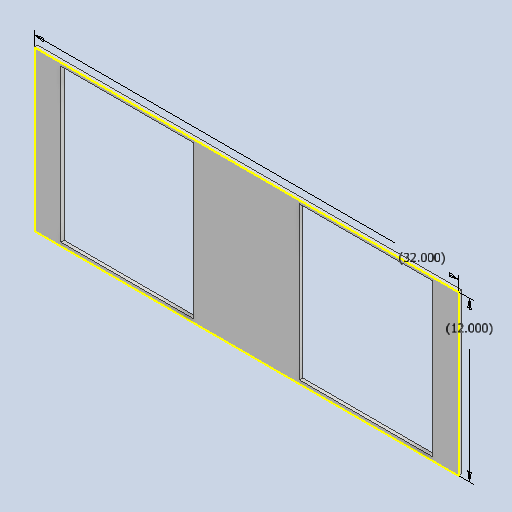
# Autodesk Inventor part: bottom_plywood_Ocampo
Saved by Autodesk Inventor 2023 (Build 270158000, 158)
## iProperties
Created: 2025-02-18
Part Number: bottom_plywood_Ocampo
Material: Generic
Document SubType Name: Modeling
Designer: 1244275
Density: 1 g/cm^3
Appearance: Default
Author: 1244275
Autodesk Inventor part; units mm, degrees
ref_plane "YZ Plane" through (0, 0, 0) normal (1, 0, 0) x (0, 1, 0)
ref_plane "XZ Plane" through (0, 0, 0) normal (0, 1, 0) x (-1, 0, 0)
ref_plane "XY Plane" through (0, 0, 0) normal (0, 0, 1) x (1, 0, 0)
sketch "Sketch1" plane through (0, 0, 0) normal (0, 0, 1) x (1, 0, 0)
  line L0 (0, 0) -> (812.8, 0)
  line L1 (812.8, 0) -> (812.8, 304.8)
  line L2 (812.8, 304.8) -> (0, 304.8)
  line L3 (0, 304.8) -> (0, 0)
  dimension "d0" = 812.8
  dimension "d1" = 304.8
  dimension "d2" = 812.8
  constraints: 8 end point, 1 horizontal, 1 perpendicular, 1 vertical
  measures "d0" distance of L0.start L0.end
  measures "d1" distance of L0.end L1.end
  measures "d2" distance of L1.end L2.end
extrude "Extrusion1" add sketch "Sketch1" along normal blind 6.35
sketch "Sketch2" plane through (0, 0, 6.35) normal (0, 0, 1) x (1, 0, 0)
  line L0 (0, 0) -> (812.8, 0) projected
  line L1 (0, 0) -> (50.8, 0)
  line L2 (50.8, 0) -> (50.8, 304.8)
  line L3 (812.8, 304.8) -> (0, 304.8) projected
  line L4 (812.8, 0) -> (762, 0)
  line L5 (762, 0) -> (762, 304.8)
  line L6 (50.8, 0) -> (50.8, 6.35)
  line L7 (50.8, 6.35) -> (304.8, 6.35)
  line L8 (50.8, 304.8) -> (50.8, 298.45)
  line L9 (50.8, 298.45) -> (304.8, 298.45)
  line L10 (304.8, 298.45) -> (304.8, 6.35)
  line L11 (50.8, 298.45) -> (50.8, 6.35)
  line L12 (0, 304.8) -> (406.4, 304.8)
  line L13 (406.4, 304.8) -> (406.4, 0)
  line L14 (406.4, 304.8) -> (406.4, -7.4745)
  line L15 (762, 6.35) -> (508, 6.35)
  line L16 (762, 298.45) -> (508, 298.45)
  line L17 (508, 298.45) -> (508, 6.35)
  line L18 (762, 298.45) -> (762, 6.35)
  point P0 (762, 6.35)
  dimension "d5" = 50.8
  dimension "d6" = 50.8
  dimension "d7" = 6.35
  dimension "d8" = 254
  dimension "d9" = 6.35
  dimension "d10" = 254
  dimension "d11" = 406.4
  constraints: 34 end point, 7 point on line, 4 symmetric about line, 3 perpendicular, 2 midpoint, 1 collinear, 1 parallel
  measures "d5" distance of L0.start L1.end
  measures "d6" distance of L0.end L4.end
  measures "d7" distance of L1.end L6.end
  measures "d8" distance of L6.end L7.end
  measures "d9" distance of L2.end L8.end
  measures "d10" distance of L8.end L9.end
  measures "d11" distance of L3.end L12.end
extrude "Extrusion2" cut sketch "Sketch2" against normal blind 57.15 contours L2 L9 L10 L7 | L15 L17 L16 L5
sketch "Sketch3" plane through (0, 0, 6.35) normal (0, 0, 1) x (1, 0, 0)
  line L0 (812.8, 0) -> (812.8, 304.8) projected
  line L1 (0, 304.8) -> (0, 0) projected
  line L2 (812.8, 304.8) -> (0, 304.8) projected
  line L3 (0, 0) -> (812.8, 0) projected
  dimension "d14" = 812.8
  dimension "d15" = 304.8
  measures "d14" distance between parallel lines of L0 L1
  measures "d15" distance between parallel lines of L2 L3
body "Solid1"
